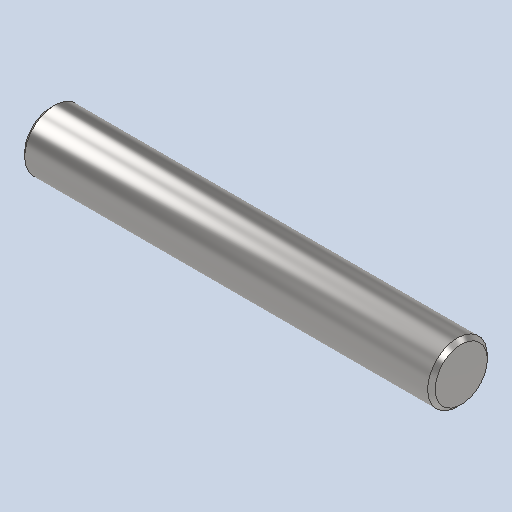
# Autodesk Inventor part: wheel_shaft_D8_V1
Saved by Autodesk Inventor 2023 (Build 270158000, 158)
## iProperties
Created: 2023-02-13
Part Number: wheel_shaft_D8_V1
Material: Stahl, Legierung
Document SubType Name: Modeling
Designer: Mathi
Density: 7.73 g/cm^3
Appearance: Halbpoliert
Author: Mathi
Autodesk Inventor part; units mm, degrees
ref_plane "YZ Plane" through (0, 0, 0) normal (1, 0, 0) x (0, 1, 0)
ref_plane "XZ Plane" through (0, 0, 0) normal (0, 1, 0) x (-1, 0, 0)
ref_plane "XY Plane" through (0, 0, 0) normal (0, 0, 1) x (1, 0, 0)
sketch "Skizze1" plane through (0, 0, 0) normal (0, 0, 1) x (1, 0, 0)
  line L0 (-41.2902, 0) -> (-18.351, 0)
  line L1 (-20, 0) -> (35, 0)
  line L2 (35, 0) -> (35, 3.5)
  line L3 (34.5, 4) -> (-19.5, 4)
  line L4 (-20, 3.5) -> (-20, 0)
  line L5 (-19.5, 4) -> (-20, 3.5)
  line L6 (35, 3.5) -> (34.5, 4)
  line L7 (-56.5482, 0) -> (50.258, 0) projected
  point P0 (0, 0)
  point P1 (35, 4)
  point P2 (-20, 4)
  dimension "d0" = 8
  dimension "d1" = 20
  dimension "d2" = 35
  dimension "d3" = 0.5
  dimension "d4" = 0.5
  dimension "d5" = 0.5
  dimension "d6" = 0.5
  constraints: 14 end point, 6 point on line, 2 horizontal, 2 parallel, 1 perpendicular
  measures "d0" diameter of L3 L0
  measures "d1" distance from line of L4 point (0, 0)
  measures "d2" distance from line of L2 point (0, 0)
  measures "d3" distance of L3.end point (-20, 4)
  measures "d4" distance of L4.start point (-20, 4)
  measures "d5" distance of L2.end point (35, 4)
  measures "d6" distance of L3.start point (35, 4)
revolve "Umdrehung1" add sketch "Skizze1" angle 360 about axis through (-10, 0, 0) along (1, 0, 0)
equation "\"d4\" = d3"
equation "\"d5\" = d3"
equation "\"d6\" = d5"
